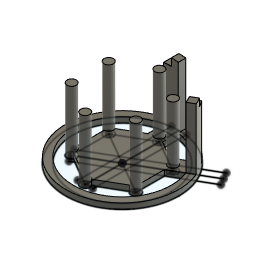
dc-15s_center_light_assembly (Autodesk Fusion 360 design; units mm, degrees)
Autodesk Fusion 360 part; units mm, degrees
sketch "Sketch1" plane through (0, 0, 0) normal (0, 1, 0) x (1, 0, 0)
  line L0 (0, -10) -> (8.6603, -5)
  line L1 (8.6603, -5) -> (8.6603, 5)
  line L2 (8.6603, 5) -> (0, 10)
  line L3 (0, 10) -> (-8.6603, 5)
  line L4 (-8.6603, 5) -> (-8.6603, -5)
  line L5 (-8.6603, -5) -> (0, -10)
  circle A0 centre (0, -10) radius 1.25
  circle A1 centre (8.6603, -5) radius 1.25
  circle A2 centre (0, 10) radius 1.25
  circle A3 centre (8.6603, 5) radius 1.25
  circle A4 centre (-8.6603, 5) radius 1.25
  circle A5 centre (-8.6603, -5) radius 1.25
  circle A6 centre (0, 0) radius 15.25
  line L6 (-8.6603, 5) -> (8.6603, -5)
  line L7 (0, 10) -> (0, -10)
  line L8 (8.6603, 5) -> (-8.6603, -5)
  line L9 (0, -10) -> (0, 15.25)
  line L10 (-8.6603, -5) -> (-8.3805, -4.5155)
  line L11 (-8.6603, -5) -> (17.3205, 10)
  line L12 (2, -10) -> (2, 15.25)
  line L13 (-2, -10) -> (-2, 15.25)
  line L14 (-7.6603, -6.7321) -> (18.3205, 8.2679)
  line L15 (-9.6603, -3.2679) -> (16.3205, 11.7321)
  circle A7 centre (0, 0) radius 13.25
  dimension "d1" = 10
  dimension "d2" = 2.5
  dimension "d3" = 2.5
  dimension "d4" = 2.5
  dimension "d5" = 2.5
  dimension "d6" = 2.5
  dimension "d7" = 2.5
  dimension "d8" = 30.5
  dimension "d9" = 30
  dimension "d10" = 2
  dimension "d11" = -2
  dimension "d12" = 2
  dimension "d13" = -2
  dimension "d14" = -2
  constraint coincident A6.centre A7.centre
  constraint coincident L0.start L5.end
  constraint coincident L0.end L1.start
  constraint coincident L2.end L3.start
  constraint coincident L1.end L2.start
  constraint coincident L3.end L4.start
  constraint coincident L4.end L5.start
  constraint vertical L7
  constraint coincident A6 L9.end
  constraint parallel L7 L9
  constraint perpendicular L5 L10
  constraint parallel L8 L11
  measures "d1" distance of L0.start A6.centre
  measures "d2" diameter of A0
  measures "d3" diameter of A1
  measures "d4" diameter of A2
  measures "d5" diameter of A3
  measures "d6" diameter of A4
  measures "d7" diameter of A5
  measures "d8" diameter of A6
  measures "d9" distance of L4.end L11.end
extrude "Extrude3" add sketch "Sketch1" along normal blind 17 contours L0 A0 L7 L9 | L0 L5 A0 | L5 A0 L7 L9 | L0 A1 L6 | L0 L1 A1 | L1 A1 L6 | L4 L5 A5 | L5 A5 L8 L11 | L1 A3 L8 L11 | L2 A3 L8 L11 | L1 A3 L11 | L4 A5 L8 L11 | L3 A4 L6 | L4 A4 L6 | L2 A2 L7 L9 | L3 A2 L7 L9 | L2 A3 L11 | L3 L4 A4 | L3 A2 L9 | L2 A2 L9 makes body 1 at (-7.4165, 5.6667, -4.8755) makes body 2 at (1.2438, 11.3333, -10.1245) makes body 3 at (9.904, 5.6667, -4.8755) makes body 4 at (1.2438, 5.6667, 10.1245) makes body 5 at (-7.4165, 5.6667, 5.1245) makes body 6 at (9.904, 11.3333, 4.8755)
extrude "Extrude2" add sketch "Sketch1" along normal blind 17 separate body contours A6 L11 L14 A7 | A6 L11 L15 A7 | A6 L9 L13 A7 | A6 L9 L12 A7 makes body 7 at (1.1141, 5.6667, -13.2031) makes body 8 at (11.3617, 11.3333, -6.8172)
extrude "Extrude1" add sketch "Sketch1" along normal blind 1.5 contours L0 A0 L7 L9 L12 L14 | L5 A0 L7 L9 L13 L14 | L0 A1 L6 L12 | L5 L13 L14 | L7 L8 L9 L11 L13 L14 | L6 L7 L9 L14 | L1 A1 L6 L14 | L6 L8 L11 L12 | L1 A3 L8 L11 L12 L14 | L5 A5 L8 L11 L13 L14 | L6 L8 L11 L13 | L6 L7 L9 L15 | L7 L8 L9 L11 L12 L15 | L2 A3 L8 L11 L12 L15 | L1 A3 L11 L14 A7 | L4 A5 L8 L11 L13 L15 | L4 A4 L6 L15 | L3 A4 L6 L13 | L3 A2 L7 L9 L13 L15 | L2 A2 L7 L9 L12 L15 | L2 L12 L15 | A6 L13 L14 A7 | L3 A2 L9 L13 A7 | L2 A3 L11 L15 A7 | L2 A2 L9 L12 A7 | A6 L12 L15 A7 bodies 2 1 3 4 5 6 7 8
sketch "Sketch2" plane through (0, 17, 0) normal (0, 1, 0) x (-1, 0, 0)
  line L0 (-2, -13.0982) -> (-2, -15.1183)
  arc A0 (-2, -15.1183) -> (2, -15.1183) centre (0, 0) ccw
  line L1 (2, -15.1183) -> (2, -13.0982)
  arc A1 (-2, -13.0982) -> (2, -13.0982) centre (0, 0) ccw
  line L2 (0, -13.25) -> (0, -15.25)
  constraint midpoint A1 L2.start
  constraint midpoint A0 L2.end
extrude "Extrude4" cut sketch "Sketch2" against normal blind 1 contours A0 L1 A1 L2 bodies 2
extrude "Extrude5" add 1 faces at (1.7787, 17, -13.7996) along direction (0, 1, 0) blind 1 on bodies 2 bodies 2
sketch "Sketch3" plane through (0, 17, 0) normal (0, 1, 0) x (-1, 0, 0)
  line L0 (-12.3434, -4.817) -> (-14.0928, -5.8271)
  arc A0 (-14.0928, -5.8271) -> (-12.0928, -9.2912) centre (0, 0) ccw
  line L1 (-12.0928, -9.2912) -> (-10.3434, -8.2811)
  arc A1 (-12.3434, -4.817) -> (-10.3434, -8.2811) centre (0, 0) ccw
  line L2 (-11.4748, -6.625) -> (-13.2069, -7.625)
  constraint midpoint A1 L2.start
  constraint midpoint A0 L2.end
extrude "Extrude6" add sketch "Sketch3" along normal blind 1 contours L0 A0 A1 L2 bodies 2
extrude "Extrude7" cut 1 faces at (11.0615, 17, -8.4402) along direction (0, -1, 0) blind 1 on bodies 2 bodies 2
named bodies: "DC-15s_Light_Assembly"
